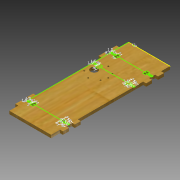
# Autodesk Inventor part: lateral_mdf
Saved by Autodesk Inventor 2014 (Build 180170000, 170)
## iProperties
Created: 2014-11-10
Part Number: lateral_mdf
Material: Generic
Document SubType Name: Modeling
Designer: Gabriel
Density: 1 g/cm^3
Appearance: Default
Author: Gabriel
Autodesk Inventor part; units mm, degrees
ref_plane "YZ Plane" through (0, 0, 0) normal (1, 0, 0) x (0, 1, 0)
ref_plane "XZ Plane" through (0, 0, 0) normal (0, 1, 0) x (-1, 0, 0)
ref_plane "XY Plane" through (0, 0, 0) normal (0, 0, 1) x (1, 0, 0)
sketch "Sketch1" plane through (0, 0, 0) normal (0, 0, 1) x (1, 0, 0)
  line L0 (0, 0) -> (70, 0)
  line L1 (70, 0) -> (70, -200)
  line L2 (70, -200) -> (0, -200)
  line L3 (0, -200) -> (0, 0)
  dimension "d0" = 70
  dimension "d1" = 200
  constraints: 8 end point, 2 parallel, 1 horizontal, 1 perpendicular
  measures "d0" distance of L1.end L2.end
  measures "d1" distance of L2.end L0.start
extrude "Extrusion1" add sketch "Sketch1" along normal blind 5
sketch "Sketch3" plane through (0, 0, 5) normal (0, 0, 1) x (1, 0, 0)
  line L0 (0, -0.5) -> (0, -3)
  line L1 (0, -3) -> (0, -30)
  line L2 (0, -3) -> (0, -2)
  line L3 (8, -1) -> (11, -1)
  line L4 (0, -30) -> (0, -28.5)
  line L5 (8, -28.5) -> (8, -26.5)
  line L6 (13, -26.5) -> (13, -33.5)
  line L7 (8, -33.5) -> (8, -31.5)
  line L8 (0, -31.5) -> (0, -30)
  line L9 (0, -30) -> (13, -30)
  line L10 (0, -30) -> (0, -60)
  line L11 (0, -60) -> (13, -60)
  line L12 (13, -60) -> (13, -56.5)
  line L13 (13, -56.5) -> (8, -56.5)
  line L14 (8, -56.5) -> (8, -58.5)
  line L15 (8, -58.5) -> (0, -58.5)
  line L16 (13, -60) -> (13, -63.5)
  line L17 (13, -63.5) -> (8, -63.5)
  line L18 (8, -63.5) -> (8, -61.5)
  line L19 (8, -61.5) -> (0, -61.5)
  line L20 (0, -60) -> (0, -90)
  line L21 (0, -90) -> (0, -170)
  line L22 (0, -170) -> (13, -170)
  line L23 (13, -170) -> (13, -166.5)
  line L24 (13, -166.5) -> (8, -166.5)
  line L25 (8, -166.5) -> (8, -168.5)
  line L26 (8, -168.5) -> (0, -168.5)
  line L27 (13, -170) -> (13, -173.5)
  line L28 (13, -173.5) -> (8, -173.5)
  line L29 (8, -173.5) -> (8, -171.5)
  line L30 (8, -171.5) -> (0, -171.5)
  line L31 (0, -171.5) -> (0, -170)
  line L32 (0, -91.5) -> (0, -90)
  line L33 (0, -61.5) -> (0, -60)
  line L34 (0, -31.5) -> (0, -30)
  line L35 (0, -4) -> (0, -3)
  line L36 (70, 0) -> (0, 0) projected
  line L37 (0, -30) -> (70, -30)
  line L38 (0, -60) -> (70, -60)
  line L39 (0, -170) -> (70, -170)
  line L40 (70, -60) -> (70, -58.5)
  line L41 (70, -58.5) -> (62, -58.5)
  line L42 (62, -58.5) -> (62, -56.5)
  line L43 (62, -56.5) -> (57, -56.5)
  line L44 (57, -56.5) -> (57, -60)
  line L45 (57, -60) -> (57, -63.5)
  line L46 (57, -63.5) -> (62, -63.5)
  line L47 (62, -63.5) -> (62, -61.5)
  line L48 (62, -61.5) -> (70, -61.5)
  line L49 (70, -61.5) -> (70, -60)
  line L50 (70, -170) -> (70, -168.5)
  line L51 (70, -168.5) -> (62, -168.5)
  line L52 (62, -168.5) -> (62, -166.5)
  line L53 (62, -166.5) -> (57, -166.5)
  line L54 (57, -166.5) -> (57, -170)
  line L55 (70, -170) -> (70, -171.5)
  line L56 (70, -171.5) -> (62, -171.5)
  line L57 (62, -171.5) -> (62, -173.5)
  line L58 (62, -173.5) -> (57, -173.5)
  line L59 (57, -173.5) -> (57, -170)
  line L60 (13, -33.5) -> (8, -33.5)
  line L61 (13, -26.5) -> (8, -26.5)
  line L62 (8, -28.5) -> (0, -28.5)
  line L63 (8, -31.5) -> (0, -31.5)
  line L64 (70, -28.5) -> (62, -28.5)
  line L65 (62, -28.5) -> (62, -26.5)
  line L66 (62, -26.5) -> (57, -26.5)
  line L67 (57, -26.5) -> (57, -30)
  line L68 (57, -30) -> (57, -33.5)
  line L69 (57, -33.5) -> (62, -33.5)
  line L70 (62, -33.5) -> (62, -31.5)
  line L71 (62, -31.5) -> (70, -31.5)
  line L72 (70, -28.5) -> (70, -30)
  line L73 (70, -30) -> (70, -31.5)
  line L74 (0, -0.5) -> (0, 0)
  dimension "d35" = 3
  dimension "d41" = 5
  dimension "d53" = 2
  dimension "d55" = 5
  dimension "d92" = 1.5
  dimension "d94" = 1.5
  dimension "d95" = 2
  dimension "d97" = 8
  dimension "d99" = 5
  dimension "d103" = 1.5
  dimension "d104" = 1.5
  dimension "d105" = 8
  dimension "d113" = 1.5
  dimension "d114" = 1.5
  dimension "d115" = 8
  dimension "d116" = 5
  dimension "d117" = 2
  dimension "d118" = 2
  dimension "d130" = 1.5
  dimension "d131" = 8
  dimension "d132" = 2
  dimension "d133" = 5
  dimension "d134" = 3.5
  dimension "d135" = 5
  dimension "d136" = 2
  dimension "d145" = 1.5
  dimension "d146" = 8
  dimension "d147" = 2
  dimension "d148" = 5
  dimension "d149" = 1.5
  dimension "d150" = 8
  dimension "d151" = 2
  dimension "d152" = 5
  constraints: 148 end point, 29 perpendicular, 27 parallel, 8 point on line, 7 collinear, 1 midpoint
  measures "d35" distance of L3.start L3.end
  measures "d41" distance of L5.end L6.start
  measures "d53" distance of L13.end L14.end
  measures "d55" distance of L16.end L17.end
  measures "d92" distance between parallel lines of L11 L15
  measures "d94" distance between parallel lines of L11 L19
  measures "d95" distance of L17.end L18.end
  measures "d97" distance of L14.end L15.end
  measures "d99" distance of L6.end L7.start
  measures "d103" distance of L8.start L1.end
  measures "d104" distance of L1.end L4.end
  measures "d105" distance of L4.end L5.start
  measures "d113" distance between parallel lines of L22 L26
  measures "d114" distance between parallel lines of L30 L22
  measures "d115" distance of L25.end L26.end
  measures "d116" distance of L23.end L24.end
  measures "d117" distance of L24.end L25.end
  measures "d118" distance of L28.end L29.end
  measures "d130" distance of L38.end L40.end
  measures "d131" distance of L40.end L41.end
  measures "d132" distance of L41.end L42.end
  measures "d133" distance of L42.end L43.end
  measures "d134" distance of L44.end L45.end
  measures "d135" distance of L45.end L46.end
  measures "d136" distance of L46.end L47.end
  measures "d145" distance of L39.end L50.end
  measures "d146" distance of L50.end L51.end
  measures "d147" distance of L51.end L52.end
  measures "d148" distance of L52.end L53.end
  measures "d149" distance of L39.end L55.end
  measures "d150" distance of L55.end L56.end
  measures "d151" distance of L56.end L57.end
  measures "d152" distance of L57.end L58.end
extrude "Extrusion3" cut sketch "Sketch3" against normal blind 5 contours L22 L27 L28 L29 L30 L31
extrude "Extrusion4" cut sketch "Sketch3" against normal blind 5 contours L26 L25 L24 L23 L22 L21
extrude "Extrusion14" cut sketch "Sketch3" against normal blind 5 contours L39 L55 L56 L57 L58 L59
extrude "Extrusion15" cut sketch "Sketch3" against normal blind 5 contours L54 L53 L52 L51 L50 L39
sketch "Sketch4" plane through (0, 0, 5) normal (0, 0, 1) x (1, 0, 0)
  line L0 (0, 0) -> (0, -19)
  circle A0 centre (11.4, -69) radius 6
  line L1 (17.4, -69) -> (34.103, -69)
  circle A1 centre (35.353, -69) radius 1.25
  line L2 (35.353, -69) -> (34.103, -69)
  line L3 (35.353, -69) -> (32.177, -69)
  line L4 (32.177, -69) -> (32.177, -78.842)
  line L5 (32.177, -69) -> (32.177, -59.158)
  circle A2 centre (32.177, -59.158) radius 1.25
  circle A3 centre (32.177, -78.842) radius 1.25
  line L6 (35.353, -69) -> (18.403, -69)
  line L7 (18.403, -69) -> (18.403, -85.95)
  line L8 (18.403, -69) -> (18.403, -52.05)
  circle A4 centre (18.403, -52.05) radius 1.25
  circle A5 centre (18.403, -85.95) radius 1.25
  line L9 (32.177, -59.158) -> (18.403, -52.05)
  line L10 (18.403, -69) -> (17.4, -69)
  line L11 (18.403, -69) -> (4.629, -69)
  line L12 (18.403, -52.05) -> (4.629, -59.158)
  circle A6 centre (4.629, -59.158) radius 1.25
  line L13 (4.629, -59.158) -> (4.629, -78.842)
  line L14 (18.403, -85.95) -> (4.629, -78.842)
  circle A7 centre (4.629, -78.842) radius 1.25
  line L15 (70, 0) -> (0, 0) projected
  dimension "d171" = 12
  dimension "d176" = 2.5
  dimension "d169" = 19
  dimension "d179" = 3.176
  dimension "d180" = 9.842
  dimension "d181" = 9.842
  dimension "d182" = 2.5
  dimension "d183" = 2.5
  dimension "d184" = 16.95
  dimension "d185" = 16.95
  dimension "d186" = 16.95
  dimension "d187" = 2.5
  dimension "d188" = 2.5
  dimension "d196" = 13.774
  dimension "d197" = 2.5
  dimension "d273" = 69
  constraints: 30 end point, 6 centre point, 6 coincident, 4 collinear, 4 point on line, 3 perpendicular, 2 horizontal alignment, 1 parallel, 1 vertical, 4 other
  measures "d169" distance of L0.start L0.end
  measures "d179" distance of L2.start L3.end
  measures "d180" distance of L3.end L4.end
  measures "d181" distance of L3.end L5.end
  measures "d182" diameter of A2
  measures "d183" diameter of A3
  measures "d184" distance of L2.start L6.end
  measures "d185" distance of L6.end L7.end
  measures "d186" distance of L6.end L8.end
  measures "d187" diameter of A4
  measures "d188" diameter of A5
  measures "d196" distance of L6.end L11.end
  measures "d197" diameter of A6
  measures "d273" distance between parallel lines of L15 L1
extrude "Extrusion22" cut sketch "Sketch4" against normal blind 5 contours L11 A0 | A0 L11
hole "Hole1" at (18.403, -85.95, 5) direction (0, 0, -1) diameter 2.5 end through all
hole "Hole2" at (4.629, -78.842, 5) at (4.629, -59.158, 5) at (4.629, -78.842, 5) direction (0, 0, -1) diameter 2.5 end through all
hole "Hole3" at (18.403, -52.05, 5) direction (0, 0, -1) diameter 2.5 end through all
hole "Hole4" at (32.177, -59.158, 5) direction (0, 0, -1) diameter 2.5 end through all
hole "Hole5" at (35.353, -69, 5) direction (0, 0, -1) diameter 2.5 end through all
hole "Hole6" at (32.177, -78.842, 5) direction (0, 0, -1) diameter 2.5 end through all
sketch "Sketch5" plane through (70, -200, 5) normal (1, 0, 0) x (0, 0, -1)
  line L0 (0, 0) -> (0, 15)
  line L1 (0, 15) -> (5, 15)
  line L2 (5, 15) -> (5, 25)
  line L3 (5, 25) -> (0, 25)
  line L4 (0, 25) -> (0, 15)
  line L5 (0, 25) -> (0, 35)
  line L6 (0, 35) -> (5, 35)
  line L7 (5, 35) -> (5, 45)
  line L8 (5, 45) -> (0, 45)
  line L9 (0, 45) -> (0, 35)
  line L10 (5, 200) -> (0, 200)
  line L11 (0, 185) -> (5, 185)
  line L12 (5, 185) -> (5, 175)
  line L13 (5, 175) -> (0, 175)
  line L14 (0, 175) -> (0, 185)
  line L15 (0, 175) -> (0, 165)
  line L16 (0, 165) -> (5, 165)
  line L17 (5, 165) -> (5, 155)
  line L18 (5, 155) -> (0, 155)
  line L19 (0, 155) -> (0, 165)
  dimension "d242" = 15
  dimension "d243" = 10
  dimension "d244" = 10
  dimension "d245" = 10
  dimension "d247" = 10
  dimension "d248" = 10
  dimension "d249" = 10
  dimension "d269" = 110
  constraints: 40 end point, 8 parallel, 6 perpendicular, 4 collinear, 1 vertical
  measures "d242" distance of L0.start L0.end
  measures "d243" distance of L1.end L2.end
  measures "d244" distance of L3.end L5.end
  measures "d245" distance of L6.end L7.end
  measures "d247" distance of L11.end L12.end
  measures "d248" distance of L13.end L15.end
  measures "d249" distance of L16.end L17.end
  measures "d269" distance between parallel lines of L8 L18
extrude "Extrusion26" add sketch "Sketch5" along normal blind 5
sketch "Sketch6" plane through (0, 0, 0) normal (-1, 0, 0) x (0, 0, 1)
  line L0 (0, 0) -> (0, -15)
  line L1 (0, -15) -> (0, -25)
  line L2 (0, -25) -> (5, -25)
  line L3 (5, -25) -> (5, -15)
  line L4 (5, -15) -> (0, -15)
  line L5 (0, -25) -> (0, -35)
  line L6 (0, -35) -> (5, -35)
  line L7 (5, -35) -> (5, -45)
  line L8 (5, -45) -> (0, -45)
  line L9 (0, -45) -> (0, -35)
  line L10 (5, -45) -> (5, -150)
  line L11 (5, -150) -> (5, -185)
  line L12 (0, -185) -> (0, -175)
  line L13 (0, -175) -> (0, -165)
  line L14 (0, -165) -> (5, -165)
  line L15 (5, -165) -> (5, -155)
  line L16 (5, -155) -> (0, -155)
  line L17 (0, -155) -> (0, -165)
  line L18 (5, -155) -> (5, -45)
  line L19 (0, -185) -> (5, -185)
  line L20 (0, -175) -> (5, -175)
  dimension "d253" = 10
  dimension "d254" = 5
  dimension "d255" = 10
  dimension "d256" = 10
  dimension "d259" = 10
  dimension "d260" = 10
  dimension "d261" = 10
  dimension "d266" = 110
  constraints: 42 end point, 7 parallel, 7 perpendicular, 4 point on line, 2 collinear, 1 vertical
  measures "d253" distance of L0.end L1.end
  measures "d254" distance of L1.end L2.end
  measures "d255" distance of L1.end L5.end
  measures "d256" distance of L6.end L7.end
  measures "d259" distance of L12.start L12.end
  measures "d260" distance of L12.end L13.end
  measures "d261" distance of L14.end L15.end
  measures "d266" distance between parallel lines of L16 L8
extrude "Extrusion28" add sketch "Sketch6" along normal blind 5 contours L4 L3 L2 L1 | L6 L7 L8 L9 | L11 L14 L17 L16 | L11 L19 L12 L20
extrude "Extrusion30" cut sketch "Sketch3" against normal blind 5 contours L62 L5 L61 L6 L9 L1 | L9 L6 L60 L7 L63 L8 | L67 L66 L65 L64 L72 L37 | L37 L73 L71 L70 L69 L68
body "Solid1"
